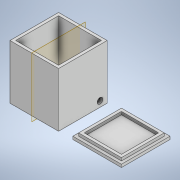
# Autodesk Inventor part: waterBallonHolderv1
Saved by Autodesk Inventor 2020.5 (Build 245400000, 400)
## iProperties
Created: 2022-09-14
Part Number: waterBallonHolderv1
Material: Generic
Document SubType Name: Modeling
Designer: kouda
Density: 1 g/cm^3
Appearance: Default
Author: kouda
Autodesk Inventor part; units mm, degrees
ref_plane "YZ Plane" through (0, 0, 0) normal (1, 0, 0) x (0, 1, 0)
ref_plane "XZ Plane" through (0, 0, 0) normal (0, 1, 0) x (-1, 0, 0)
ref_plane "XY Plane" through (0, 0, 0) normal (0, 0, 1) x (1, 0, 0)
sketch "Sketch1" plane through (0, 0, 0) normal (0, 1, 0) x (-1, 0, 0)
  line L0 (0, 0) -> (-34, 0)
  line L1 (-34, 0) -> (-34, 34)
  line L2 (-34, 34) -> (0, 34)
  line L3 (0, 34) -> (0, 0)
  dimension "d0" = 34
  dimension "d1" = 34
  constraints: 8 end point, 2 parallel, 1 horizontal, 1 perpendicular
  measures "d0" distance of L1.end L2.end
  measures "d1" distance of L0.end L1.end
extrude "Extrusion1" add sketch "Sketch1" along normal blind 38
sketch "Sketch2" plane through (0, 38, 0) normal (0, 1, 0) x (1, 0, 0)
  line L0 (0, -34) -> (34, -34) projected
  line L1 (34, -34) -> (34, 0) projected
  line L2 (34, 0) -> (0, 0) projected
  line L3 (0, 0) -> (0, -34) projected
  line L4 (2, -2) -> (32, -2)
  line L5 (32, -2) -> (32, -32)
  line L6 (32, -32) -> (2, -32)
  line L7 (2, -32) -> (2, -2)
  dimension "d4" = 2
  constraints: 8 end point, 3 other
  measures "d4" distance between parallel lines of L2 L4
extrude "Extrusion2" cut sketch "Sketch2" against normal blind 36 contours L4 L5 L6 L7
sketch "Sketch3" plane through (34, 0, 34) normal (1, 0, 0) x (0, 0, -1)
  line L0 (0, 0) -> (34, 0) projected
  line L1 (34, 0) -> (34, 38) projected
  line L2 (0, 38) -> (34, 38) projected
  line L3 (0, 0) -> (0, 38) projected
  line L4 (2, 38) -> (32, 38) projected
  line L5 (2, 38) -> (2, 2) projected
  line L6 (2, 2) -> (32, 2) projected
  line L7 (32, 38) -> (32, 2) projected
  line L8 (34, 0) -> (34, 38) projected
  line L9 (34, 0) -> (29, 0)
  line L10 (0, 0) -> (34, 0) projected
  line L11 (29, 0) -> (29, 4)
  dimension "d7" = 5
  dimension "d8" = 4
  constraints: 4 end point, 1 coincident, 1 perpendicular, 1 point on line
  measures "d7" distance of L8.start L9.end
  measures "d8" distance of L9.end L11.end
hole "Hole1" at (34, 4, 5) direction (-1, 0, 0) diameter 4 depth 2 tip angle 118
ref_plane "Work Plane1" through (17, 38, 32) normal (1, 0, 0) x (0, 0, -1)
mirror "Mirror1" about plane through (17, 38, 32) normal (1, 0, 0) of "Hole1"
sketch "Sketch4" plane through (0, 0, 0) normal (0, 1, 0) x (-1, 0, 0)
  line L0 (-34, 34) -> (-34, 0) projected
  line L1 (-34, 0) -> (-44, 0)
  line L2 (-44, 0) -> (-78, 0)
  line L3 (-78, 0) -> (-78, 34)
  line L4 (-78, 34) -> (-44, 34)
  line L5 (-44, 34) -> (-44, 0)
  point P0 (0, 0)
  dimension "d16" = 10
  dimension "d17" = 34
  dimension "d18" = 34
  constraints: 10 end point, 2 horizontal, 2 parallel, 1 perpendicular
  measures "d16" distance of L0.end L1.end
  measures "d17" distance of L3.end L4.end
  measures "d18" distance of L2.end L3.end
extrude "Extrusion3" add sketch "Sketch4" along normal blind 2
sketch "Sketch5" plane through (0, 2, 0) normal (0, 1, 0) x (1, 0, 0)
  line L0 (44, 0) -> (44, -34) projected
  line L1 (44, -34) -> (78, -34) projected
  line L2 (78, -34) -> (78, 0) projected
  line L3 (78, 0) -> (44, 0) projected
  line L4 (46, -2) -> (46, -32)
  line L5 (46, -32) -> (76, -32)
  line L6 (76, -32) -> (76, -2)
  line L7 (76, -2) -> (46, -2)
  line L8 (48, -4) -> (48, -30)
  line L9 (48, -30) -> (74, -30)
  line L10 (74, -30) -> (74, -4)
  line L11 (74, -4) -> (48, -4)
  point P0 (0, 0)
  dimension "d21" = 2
  dimension "d22" = 2
  constraints: 16 end point, 6 other
  measures "d21" distance between parallel lines of L3 L7
  measures "d22" distance between parallel lines of L7 L11
extrude "Extrusion4" add sketch "Sketch5" along normal blind 2 contours L7 L6 L5 L4
body "Solid1"
